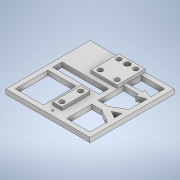
# Autodesk Inventor part: HallSensor_Halterung
Saved by Autodesk Inventor 2022.2 (Build 262287010, 287A)
## iProperties
Created: 2024-01-10
Part Number: HallSensor_Halterung
Material: Generisch
Document SubType Name: Modeling
Designer: ppovolni
Density: 1 g/cm^3
Appearance: Vorgabe
Author: ppovolni
Autodesk Inventor part; units mm, degrees
ref_plane "YZ Plane" through (0, 0, 0) normal (1, 0, 0) x (0, 1, 0)
ref_plane "Arbeitsebene1" through (-75, 27.1, 0) normal (0, 0, 1) x (0, 1, 0)
sketch "center1" plane through (-75, 27.1, 0) normal (0, 0, 1) x (0, 1, 0)
  line L0 (-173.891, -75) -> (168.1592, -75)
  line L1 (0, 239.86) -> (0, -220.81)
  point P0 (-27.1, -75)
  constraints: 4 end point, 1 horizontal, 1 vertical, 4 other
ref_plane "Arbeitsebene2" through (0, 99.4, -2.4) normal (-1, 0, 0) x (0, 0, 1)
sketch "center2" plane through (0, 99.4, -2.4) normal (-1, 0, 0) x (0, 0, 1)
  line L0 (184.8129, -72.3) -> (-258.9785, -72.3)
  point P0 (2.4, -99.4)
  constraints: 2 end point, 1 horizontal, 2 other
sketch "Hallsens" plane through (0, 0, 0) normal (0, 1, 0) x (-1, 0, 0)
  line L0 (406.994, 0) -> (-237.944, 0) construction
  line L1 (0, -350.1368) -> (0, 271.1712) construction
  line L2 (-5, 0) -> (5, 0) construction
  line L3 (5, 0) -> (5, -20) construction
  line L4 (5, -20) -> (-5, -20) construction
  line L5 (-5, -20) -> (-5, 0) construction
  line L6 (-4, -1) -> (-6, -1)
  line L7 (-6, -1) -> (-6, 1)
  line L8 (-6, 1) -> (-4, 1)
  line L9 (-4, 1) -> (-4, -1)
  line L10 (-4, -1) -> (-6, 1) construction
  line L11 (-6, -1) -> (-4, 1) construction
  line L12 (4, -1) -> (6, -1)
  line L13 (6, -1) -> (6, 1)
  line L14 (6, 1) -> (4, 1)
  line L15 (4, 1) -> (4, -1)
  line L16 (4, -1) -> (6, 1) construction
  line L17 (6, -1) -> (4, 1) construction
  line L18 (4, -21) -> (6, -21)
  line L19 (6, -21) -> (6, -19)
  line L20 (6, -19) -> (4, -19)
  line L21 (4, -19) -> (4, -21)
  line L22 (4, -21) -> (6, -19) construction
  line L23 (6, -21) -> (4, -19) construction
  line L24 (-6, -21) -> (-4, -21)
  line L25 (-4, -21) -> (-4, -19)
  line L26 (-4, -19) -> (-6, -19)
  line L27 (-6, -19) -> (-6, -21)
  line L28 (-6, -21) -> (-4, -19) construction
  line L29 (-4, -21) -> (-6, -19) construction
  line L30 (-9, 10) -> (9, 10) construction
  line L31 (9, 10) -> (9, -40) construction
  line L32 (9, -40) -> (-9, -40) construction
  line L33 (-9, -40) -> (-9, 10) construction
  circle A0 centre (0, 10) radius 1.6
  circle A1 centre (9, -40) radius 1.6
  circle A2 centre (-9, -40) radius 1.6
  dimension "d126" = 10
  dimension "d127" = 20
  dimension "d128" = 5
  dimension "d129" = 2
  dimension "d130" = 4
  dimension "d131" = 4
  dimension "d132" = 10
  dimension "d133" = 20
  dimension "d134" = 3.2
  constraints: 64 end point, 12 parallel, 9 midpoint, 7 equal length, 6 horizontal, 6 perpendicular, 3 centre point, 2 coincident, 2 equal radius, 2 point on line
  measures "d126" distance of L3.end L4.end
  measures "d127" distance of L4.end L2.start
  measures "d128" distance between parallel lines of L3 L1
  measures "d129" distance of L7.end L8.end
  measures "d130" distance between parallel lines of L31 L3
  measures "d131" distance between parallel lines of L33 L5
  measures "d132" distance between parallel lines of L0 L30
  measures "d133" distance between parallel lines of L32 L4
  measures "d134" diameter of A0
sketch "Groundplane" plane through (0, 0, 0) normal (0, 1, 0) x (-1, 0, 0)
  line L0 (45, 45) -> (-45, 45) construction
  line L1 (-45, 45) -> (-45, -45) construction
  line L2 (-45, -45) -> (45, -45) construction
  line L3 (45, -45) -> (45, 45) construction
  line L4 (1, 45) -> (-1, 45) construction
  line L5 (-1, 45) -> (-1, 40) construction
  line L6 (-1, 40) -> (1, 40) construction
  line L7 (1, 40) -> (1, 45) construction
  arc A0 (-1, 40) -> (1, 40) centre (0, 40) ccw construction
  line L8 (1, -45) -> (-1, -45) construction
  line L9 (-1, -45) -> (-1, -40) construction
  line L10 (-1, -40) -> (1, -40) construction
  line L11 (1, -40) -> (1, -45) construction
  arc A1 (1, -40) -> (-1, -40) centre (0, -40) ccw construction
  point P0 (0, 0)
  dimension "d5" = 2
  dimension "d6" = 5
  dimension "d7" = 2
  dimension "d8" = 5
  dimension "d9" = 90
  dimension "d89" = 45
  dimension "d90" = 45
  constraints: 24 end point, 6 parallel, 4 perpendicular, 4 point on circle, 3 horizontal, 2 centre point, 2 point on line, 2 tangent, 2 vertical alignment, 1 midpoint
  measures "d5" distance between parallel lines of L5 L7
  measures "d6" distance of L4.end L5.end
  measures "d7" distance between parallel lines of L9 L11
  measures "d8" distance of L8.end L9.end
  measures "d9" distance of L2.end L0.start
  measures "d89" distance from line of L0 point (0, 0)
  measures "d90" distance from line of point (0, 0) L1
sketch "Montagepunkte" plane through (0, 0, 0) normal (0, 1, 0) x (-1, 0, 0)
  circle A0 centre (0, 10) radius 1.6 projected
  circle A1 centre (9, -40) radius 1.6 projected
  circle A2 centre (-9, -40) radius 1.6 projected
  arc A3 (1, -40) -> (-1, -40) centre (0, -40) ccw construction
  arc A4 (-1, 40) -> (1, 40) centre (0, 40) ccw construction
  circle A5 centre (0, 40) radius 1
  circle A6 centre (0, -40) radius 1
  line L0 (-9, -40) -> (9, -40) construction
  line L1 (9, -40) -> (9, -20) construction
  line L2 (9, -20) -> (-9, -20) construction
  line L3 (-9, -20) -> (-9, -40) construction
  line L4 (0, 10) -> (0, 30) construction
  circle A7 centre (9, -20) radius 1.6
  circle A8 centre (-9, -20) radius 1.6
  circle A9 centre (0, 30) radius 1.6
  dimension "d135" = 2
  dimension "d136" = 20
  dimension "d137" = 20
  dimension "d138" = 3.2
  constraints: 10 end point, 5 centre point, 5 coincident, 3 equal radius, 2 parallel, 1 horizontal, 1 perpendicular, 1 point on line, 1 vertical
  measures "d135" diameter of A5
  measures "d136" distance of L2.end L0.start
  measures "d137" distance of L4.start L4.end
  measures "d138" diameter of A9
sketch "Skizze5" plane through (0, 0, 0) normal (0, 1, 0) x (-1, 0, 0)
  line L0 (45, 45) -> (-45, 45) projected
  line L1 (-45, 45) -> (-45, -45) projected
  line L2 (-45, -45) -> (45, -45) projected
  line L3 (45, -45) -> (45, 45) projected
  circle A0 centre (0, 40) radius 1 projected
  circle A1 centre (0, -40) radius 1 projected
extrude "Extrusion2" add sketch "Skizze5" along normal blind 5
sketch "Skizze6" plane through (0, 5, 0) normal (0, 1, 0) x (1, 0, 0)
  line L0 (-5, -5) -> (5, -5)
  line L1 (5, -5) -> (5, -35)
  line L2 (5, -35) -> (-5, -35)
  line L3 (-5, -35) -> (-5, -5)
  line L4 (-14, 45) -> (14, 45)
  line L5 (14, 45) -> (14, 15)
  line L6 (14, 15) -> (-14, 15)
  line L7 (-14, 15) -> (-14, 45)
  circle A0 centre (0, -40) radius 1 projected
  circle A1 centre (0, -40) radius 1 projected
  circle A2 centre (0, -30) radius 1.6 projected
  circle A3 centre (0, -10) radius 1.6 projected
  circle A4 centre (-9, 20) radius 1.6 projected
  circle A5 centre (9, 20) radius 1.6 projected
  circle A6 centre (9, 40) radius 1.6 projected
  circle A7 centre (-9, 40) radius 1.6 projected
  circle A8 centre (0, 40) radius 1 projected
  point P0 (0, 0)
  dimension "d139" = 5
  dimension "d140" = 5
  dimension "d141" = 5
  dimension "d142" = 5
  dimension "d143" = 5
  dimension "d144" = 5
  dimension "d145" = 5
  dimension "d146" = 5
  constraints: 16 end point, 4 parallel, 2 horizontal, 2 perpendicular
  measures "d139" distance from line of A2.centre L2
  measures "d140" distance from line of L0 A3.centre
  measures "d141" distance from line of L1 A3.centre
  measures "d142" distance from line of L3 A3.centre
  measures "d143" distance from line of A5.centre L6
  measures "d144" distance from line of A4.centre L7
  measures "d145" distance from line of L4 A7.centre
  measures "d146" distance from line of A6.centre L5
extrude "Extrusion3" add sketch "Skizze6" along normal blind 3 contours L0 L1 L2 L3 | L4 L5 L6 L7
chamfer "Fase1" distance 1 distance2 3 4 edges at (7.4, 8, -20) (-10.6, 8, -20) (-10.6, 8, -40) (7.4, 8, -40) measured on face at (0.0402, 8, -27.0431)
chamfer "Fase2" distance 1 distance2 3 2 edges at (-1.6, 8, 30) (-1.6, 8, 10) measured on face at (3.8056, 8, 16.9145)
sketch "Skizze8" plane through (0, 8, 0) normal (0, 1, 0) x (1, 0, 0)
  circle A0 centre (0, 40) radius 3
  circle A1 centre (0, 40) radius 1 projected
  circle A2 centre (0, 40) radius 1 projected
  circle A3 centre (0, 40) radius 1 projected
  point P0 (0, 0)
  dimension "d99" = 6
  constraints: 1 centre point, 1 coincident
  measures "d99" diameter of A0
extrude "Extrusion5" cut sketch "Skizze8" against normal up to surface (3 mm away) contours A0 | A1
sketch "Skizze9" plane through (0, 5, 0) normal (0, 1, 0) x (1, 0, 0)
  line L0 (15, 40) -> (40, 40)
  line L1 (40, 40) -> (40, -40)
  line L2 (40, -40) -> (15, -40)
  line L3 (15, -40) -> (15, 40)
  line L4 (15, 40) -> (15, -40) construction
  line L5 (31, 28) -> (31, 18)
  line L6 (31, 25) -> (15, 25)
  line L7 (31, 21) -> (15, 21)
  line L8 (15, 21) -> (15, 25)
  line L9 (31, 28) -> (41, 24.4341)
  line L10 (41, 24.4341) -> (41, 21.5659)
  line L11 (41, 21.5659) -> (31, 18)
  line L12 (-40, 10) -> (10, 10)
  line L13 (10, 10) -> (10, 0)
  line L14 (10, 0) -> (-40, 0)
  line L15 (-40, 0) -> (-40, 10)
  line L16 (-40, -5) -> (-10, -5)
  line L17 (-10, -5) -> (-10, -40)
  line L18 (-10, -40) -> (-40, -40)
  line L19 (-40, -40) -> (-40, -5)
  line L20 (-5, -5) -> (-5, -35) projected
  line L21 (-14, 15) -> (14, 15) projected
  line L22 (5, -5) -> (-5, -5) projected
  line L23 (-45, -45) -> (45, -45) construction
  line L24 (45, -45) -> (45, 45) construction
  line L25 (45, 45) -> (14, 45) construction
  line L26 (-14, 45) -> (-45, 45) construction
  line L27 (-45, 45) -> (-45, -45) construction
  point P0 (0, 0)
  point P1 (9, 45)
  point P2 (40, 23)
  point P3 (31, 23)
  point P4 (41, 23)
  point P5 (40, 21.2093)
  point P6 (40, 24.7907)
  point P7 (-40, -22.5)
  dimension "d106" = 25
  dimension "d107" = 0
  dimension "d108" = 3
  dimension "d109" = 3
  dimension "d110" = 4
  dimension "d111" = 9
  dimension "d112" = 15
  dimension "d115" = 1
  dimension "d118" = 5
  dimension "d119" = 5
  dimension "d123" = 5
  dimension "d124" = 5
  dimension "d125" = 5
  dimension "d147" = 5
  dimension "d148" = 5
  dimension "d149" = 5
  dimension "d150" = 5
  dimension "d151" = 5
  dimension "d152" = 5
  constraints: 40 end point, 7 point on line, 6 parallel, 5 perpendicular, 4 vertical, 3 horizontal, 3 midpoint, 2 horizontal alignment, 1 collinear
  measures "d106" distance of L1.end L2.end
  measures "d107" distance between parallel lines of L3 L4
  measures "d108" distance of L6.start L5.start
  measures "d109" distance of L5.end L7.start
  measures "d110" distance between parallel lines of L7 L6
  measures "d111" distance from line of point (40, 23) L5
  measures "d112" distance between parallel lines of L6 L0
  measures "d115" distance between parallel lines of L1 L10
  measures "d118" distance between parallel lines of L16 L14
  measures "d119" distance between parallel lines of L3 L13
  measures "d123" distance between parallel lines of L17 L20
  measures "d124" distance between parallel lines of L21 L12
  measures "d125" distance between parallel lines of L22 L14
  measures "d147" distance between parallel lines of L2 L23
  measures "d148" distance between parallel lines of L18 L23
  measures "d149" distance between parallel lines of L27 L19
  measures "d150" distance between parallel lines of L27 L15
  measures "d151" distance between parallel lines of L24 L1
  measures "d152" distance between parallel lines of L25 L0
extrude "Extrusion6" cut sketch "Skizze9" against normal through all contours L0 L1 L9 L5 L6 L3 | L7 L5 L11 L1 L2 L3 | L12 L13 L14 L15 | L16 L17 L18 L19
sketch "Skizze10" plane through (0, 5, 0) normal (0, 1, 0) x (1, 0, 0)
  line L0 (15, -40) -> (15, 21) construction
  line L1 (42, 2.9607) -> (26.2682, -6.3602)
  line L2 (26.2682, -6.3602) -> (15, -6.3602)
  line L3 (15, -6.3602) -> (15, -13.143)
  line L4 (15, -13.143) -> (25.94, -13.143)
  line L5 (25.94, -13.143) -> (42, -22.6171)
  line L6 (42, -22.6171) -> (42, -14.8934)
  line L7 (42, -14.8934) -> (32.3728, -9.6203)
  line L8 (32.3728, -9.6203) -> (42, -4.5223)
  line L9 (42, -4.5223) -> (42, 2.9607)
  point P0 (0, 0)
  constraints: 1 vertical
extrude "Extrusion7" add sketch "Skizze10" against normal up to surface (5 mm away)
